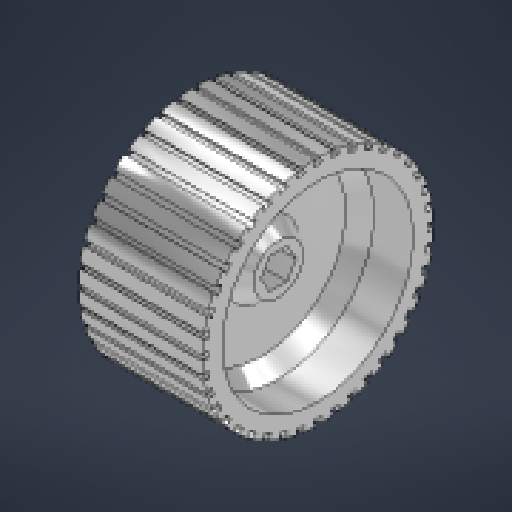
# Autodesk Inventor part: PLATE,FLYWHEEL,HUB
Saved by Autodesk Inventor 2026.1 (Build 301233020, 233B)
## iProperties
Created: 2026-02-01
Part Number: PLATE,FLYWHEEL,HUB
Material: Aluminum 6061
Document SubType Name: Modeling
Designer: Owen L
Mass: 364.842 g
Surface Area: 524.527 cm^2
Volume: 135.127 cm^3
Density: 2.7 g/cm^3
Appearance: Aluminum - Flat
Author: Owen L
Autodesk Inventor part; units mm, degrees
ref_plane "YZ Plane" through (0, 0, 0) normal (1, 0, 0) x (0, 1, 0)
ref_plane "XZ Plane" through (0, 0, 0) normal (0, 1, 0) x (-1, 0, 0)
ref_plane "XY Plane" through (0, 0, 0) normal (0, 0, 1) x (1, 0, 0)
sketch "Sketch1" plane through (0, 0, 0) normal (0, 0, 1) x (1, 0, 0)
  line L0 (0, -9.525) -> (0, 57.15) projected
  line L1 (-35.56, 0) -> (35.56, 0) projected
  line L2 (-9.1948, 0) -> (-9.1948, 10.16)
  line L3 (-9.1948, 10.16) -> (-2.3813, 14.9309)
  line L4 (-2.3813, 14.9309) -> (-2.3813, 34.5991)
  line L5 (-2.3813, 34.5991) -> (-9.1948, 39.37)
  line L6 (-9.1948, 39.37) -> (-25.4, 39.37)
  line L7 (-25.4, 39.37) -> (-25.4, 47.625)
  line L8 (-25.4, 47.625) -> (0, 47.625)
  line L9 (9.1948, 0) -> (9.1948, 10.16)
  line L10 (9.1948, 10.16) -> (2.3813, 14.9309)
  line L11 (2.3813, 14.9309) -> (2.3813, 34.5991)
  line L12 (2.3813, 34.5991) -> (9.1948, 39.37)
  line L13 (9.1948, 39.37) -> (25.4, 39.37)
  line L14 (25.4, 39.37) -> (25.4, 47.625)
  line L15 (25.4, 47.625) -> (0, 47.625)
  point P0 (0, 0)
  dimension "d0" = 10.16
  dimension "d1" = 18.3896
  dimension "d3" = 4.7625
  dimension "d4" = 35
  dimension "d5" = 35
  dimension "d6" = 50.8
  dimension "d7" = 8.255
  dimension "d8" = 95.25
  constraints: 28 end point, 7 symmetric about line, 3 perpendicular, 2 point on line, 2 vertical, 1 equal length
  measures "d0" distance of L2.start L2.end
  measures "d1" diameter of L2 L0
  measures "d3" diameter of L4 L0
  measures "d4" angle of L1 L3
  measures "d5" angle of L5 L1
  measures "d6" diameter of L7 L0
  measures "d7" distance of L6.end L7.end
  measures "d8" diameter of L8 L1
revolve "Revolution1" add sketch "Sketch1" angle 360 about axis through (-10, 0, 0) along (1, 0, 0)
sketch "Sketch2" plane through (-9.1948, 0, 0) normal (-1, 0, 0) x (0, 0, 1)
  circle A0 centre (0, 0) radius 14.9309 projected
  line L0 (7.3323, 0) -> (3.6662, -6.35)
  line L1 (3.6662, -6.35) -> (-3.6662, -6.35)
  line L2 (-3.6662, -6.35) -> (-7.3323, 0)
  line L3 (-7.3323, 0) -> (-3.6662, 6.35)
  line L4 (-3.6662, 6.35) -> (3.6662, 6.35)
  line L5 (3.6662, 6.35) -> (7.3323, 0)
  dimension "d10" = 12.7
  constraints: 12 end point, 1 coincident, 1 horizontal, 13 other
  measures "d10" distance between parallel lines of L4 L1
extrude "Extrusion1" cut sketch "Sketch2" against normal through all contours L0 L1 L2 L3 L4 L5
sketch "Sketch3" plane through (-25.4, 0, 0) normal (-1, 0, 0) x (0, 0, 1)
  circle A0 centre (0, 0) radius 47.625 projected
  line L0 (-1.016, 47.6142) -> (-2.0955, 45.212)
  line L1 (1.016, 47.6142) -> (2.0955, 45.212)
  line L2 (2.0955, 45.212) -> (-2.0955, 45.212)
  point P0 (0, 45.212)
  dimension "d13" = 4.191
  dimension "d14" = 2.413
  dimension "d15" = 2.032
  constraints: 6 end point, 2 point on circle, 1 equal length, 1 horizontal, 1 midpoint, 1 vertical alignment
  measures "d13" distance of L1.end L0.end
  measures "d14" distance edge to line of A0 L2
  measures "d15" distance of L1.start L0.start
extrude "Extrusion2" cut sketch "Sketch3" against normal through all contours L1 L2 L0 A0 picked at (0.1129, 46.0159)
fillet "Fillet1" radius 0.508 2 edges at (0, 45.212, 2.0955) (0, 45.212, -2.0955)
pattern_circular "Circular Pattern1" count 40 over 360 about axis through (0, 0, 0) along (1, 0, 0) of "Extrusion2", "Fillet1"
body "Solid1"
